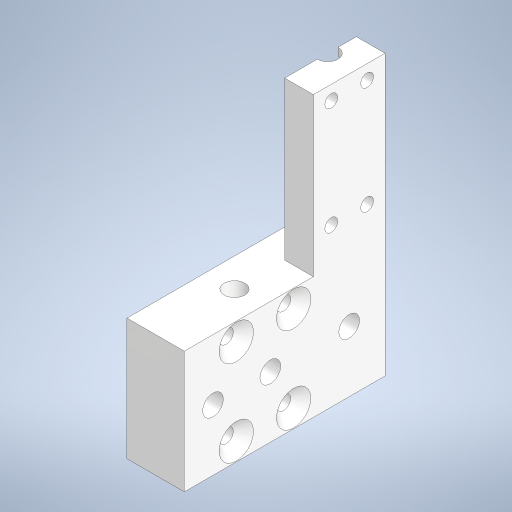
# Autodesk Inventor part: Z_probe_holder
Saved by Autodesk Inventor 2024.1 (Build 281209000, 209)
## iProperties
Created: 2023-10-06
Part Number: Z_probe_holder
Material: Generic
Document SubType Name: Modeling
Designer: l1534
Density: 1 g/cm^3
Appearance: White
Author: l1534
Autodesk Inventor part; units mm, degrees
ref_plane "YZ Plane" through (0, 0, 0) normal (1, 0, 0) x (0, 1, 0)
ref_plane "XZ Plane" through (0, 0, 0) normal (0, 1, 0) x (-1, 0, 0)
ref_plane "XY Plane" through (0, 0, 0) normal (0, 0, 1) x (1, 0, 0)
sketch "Sketch1" plane through (0, 0, 0) normal (1, 0, 0) x (0, 1, 0)
  line L0 (3.2139, -35.6679) -> (20.2139, -35.6679)
  line L1 (20.2139, -35.6679) -> (20.2139, -63.6679)
  line L2 (20.2139, -63.6679) -> (3.2139, -63.6679)
  line L3 (3.2139, -63.6679) -> (3.2139, -35.6679)
  point P0 (0, 0)
  dimension "d0" = 17
  dimension "d1" = 28
  constraints: 8 end point, 2 parallel, 1 horizontal, 1 perpendicular
  measures "d0" distance of L0.start L0.end
  measures "d1" distance of L0.end L1.end
extrude "Extrusion1" add sketch "Sketch1" along normal blind 8
sketch "Sketch2" plane through (8, 0, 0) normal (1, 0, 0) x (0, 0, -1)
  line L0 (63.6679, 3.2139) -> (63.6679, 20.2139) projected
  line L1 (63.6679, 20.2139) -> (53.6679, 20.2139)
  line L2 (53.6679, 20.2139) -> (53.6679, 42.2139)
  line L3 (53.6679, 42.2139) -> (63.6679, 42.2139)
  line L4 (63.6679, 42.2139) -> (63.6679, 20.2139)
  point P0 (0, 0)
  dimension "d4" = 10
  dimension "d5" = 22
  constraints: 8 end point, 2 parallel, 1 horizontal, 1 perpendicular
  measures "d4" distance of L2.end L3.end
  measures "d5" distance of L1.end L2.end
extrude "Extrusion2" add sketch "Sketch2" against normal up to surface (8 mm away)
sketch "Sketch3" plane through (8, 20.2139, -53.6679) normal (0, 0, 1) x (1, 0, 0)
  line L0 (-8, 0) -> (0, 0) projected
  line L1 (-8, -17) -> (-8, 22) projected
  line L2 (-4, 0) -> (-8, 0)
  line L3 (-8, 0) -> (-8, 22)
  line L4 (-8, 22) -> (-4, 22)
  line L5 (-4, 22) -> (-4, 0)
  point P0 (-8, -20.2139)
  dimension "d8" = 4
  constraints: 8 end point, 2 parallel, 1 horizontal, 1 midpoint, 1 perpendicular
  measures "d8" distance between parallel lines of L1 L5
extrude "Extrusion3" cut sketch "Sketch3" against normal through all
sketch "Sketch4" plane through (8, 0, 0) normal (1, 0, 0) x (0, 0, -1)
  circle A0 centre (42.9179, 5.7139) radius 1
  circle A1 centre (42.9179, 17.7139) radius 1
  circle A2 centre (50.9179, 5.7139) radius 1
  circle A3 centre (50.9179, 17.7139) radius 1
  line L0 (35.6679, 3.2139) -> (63.6679, 3.2139) projected
  line L1 (53.6679, 20.2139) -> (35.6679, 20.2139) projected
  line L2 (35.6679, 20.2139) -> (35.6679, 3.2139) projected
  point P0 (0, 0)
  dimension "d11" = 2
  dimension "d13" = 2
  dimension "d14" = 2
  dimension "d15" = 2
  dimension "d16" = 2.5
  dimension "d17" = 2.5
  dimension "d18" = 2.5
  dimension "d19" = 2.5
  dimension "d20" = 7.25
  dimension "d21" = 7.25
  dimension "d22" = 8
  dimension "d23" = 8
  constraints: 4 centre point
  measures "d11" diameter of A2
  measures "d13" diameter of A1
  measures "d14" diameter of A3
  measures "d15" diameter of A0
  measures "d16" distance from line of L0 A0.centre
  measures "d17" distance from line of L1 A1.centre
  measures "d18" distance from line of L1 A3.centre
  measures "d19" distance from line of L0 A2.centre
  measures "d20" distance from line of L2 A0.centre
  measures "d21" distance from line of L2 A1.centre
  measures "d22" distance of A0.centre A2.centre
  measures "d23" distance of A1.centre A3.centre
extrude "Extrusion4" cut sketch "Sketch4" against normal through all
sketch "Sketch5" plane through (0, 3.2139, -63.6679) normal (0, -1, 0) x (1, 0, 0)
  line L0 (4, 10) -> (4, 0) projected
  circle A0 centre (4, 4) radius 1.45
  circle A1 centre (4, 17) radius 1.45
  line L1 (8, 28) -> (8, 0) projected
  line L2 (0, 0) -> (8, 0) projected
  point P0 (0, 63.6679)
  dimension "d26" = 2.9
  dimension "d27" = 2.9
  dimension "d28" = 4
  dimension "d29" = 4
  dimension "d30" = 17
  constraints: 2 centre point, 1 point on line
  measures "d26" diameter of A1
  measures "d27" diameter of A0
  measures "d28" distance from line of L1 A1.centre
  measures "d29" distance from line of L2 A0.centre
  measures "d30" distance from line of L2 A1.centre
extrude "Extrusion5" cut sketch "Sketch5" against normal through all
chamfer "Chamfer1" distance 0.2 angle 45 2 edges at (2.55, 3.2139, -46.6679) (2.55, 3.2139, -59.6679)
sketch "Sketch7" plane through (8, 0, 0) normal (1, 0, 0) x (0, 0, -1)
  circle A0 centre (56.1679, 25.2139) radius 0.9
  circle A1 centre (56.1679, 40.2139) radius 0.9
  circle A2 centre (61.1679, 25.2139) radius 0.9
  circle A3 centre (61.1679, 40.2139) radius 0.9
  line L0 (53.6679, 42.2139) -> (53.6679, 20.2139) projected
  line L1 (63.6679, 3.2139) -> (63.6679, 42.2139) projected
  line L2 (63.6679, 42.2139) -> (53.6679, 42.2139) projected
  point P0 (0, 0)
  dimension "d36" = 1.8
  dimension "d37" = 1.8
  dimension "d38" = 1.8
  dimension "d39" = 1.8
  dimension "d40" = 2.5
  dimension "d41" = 2.5
  dimension "d42" = 2.5
  dimension "d43" = 2.5
  dimension "d44" = 15
  dimension "d45" = 15
  dimension "d46" = 2
  dimension "d47" = 2
  constraints: 4 centre point
  measures "d36" diameter of A0
  measures "d37" diameter of A2
  measures "d38" diameter of A1
  measures "d39" diameter of A3
  measures "d40" distance from line of L0 A0.centre
  measures "d41" distance from line of L1 A2.centre
  measures "d42" distance from line of L0 A1.centre
  measures "d43" distance from line of L1 A3.centre
  measures "d44" distance of A3.centre A2.centre
  measures "d45" distance of A1.centre A0.centre
  measures "d46" distance from line of L2 A1.centre
  measures "d47" distance from line of L2 A3.centre
extrude "Extrusion6" cut sketch "Sketch7" against normal through all
sketch "Sketch8" plane through (8, 0, 0) normal (1, 0, 0) x (0, 0, -1)
  circle A0 centre (39.6679, 11.7139) radius 1.45
  circle A1 centre (58.6679, 11.7139) radius 1.45
  circle A2 centre (47.6679, 11.7139) radius 1.45
  line L0 (53.6679, 20.2139) -> (35.6679, 20.2139) projected
  line L1 (35.6679, 3.2139) -> (63.6679, 3.2139) projected
  line L2 (63.6679, 3.2139) -> (63.6679, 42.2139) projected
  line L3 (35.6679, 20.2139) -> (35.6679, 3.2139) projected
  point P0 (0, 0)
  dimension "d53" = 8.5
  dimension "d54" = 8.5
  dimension "d55" = 8.5
  dimension "d56" = 2.9
  dimension "d57" = 2.9
  dimension "d58" = 2.9
  dimension "d59" = 5
  dimension "d60" = 16
  dimension "d61" = 4
  constraints: 3 centre point
  measures "d53" distance from line of L0 A0.centre
  measures "d54" distance from line of L0 A2.centre
  measures "d55" distance from line of L1 A1.centre
  measures "d56" diameter of A0
  measures "d57" diameter of A2
  measures "d58" diameter of A1
  measures "d59" distance from line of L2 A1.centre
  measures "d60" distance from line of L2 A2.centre
  measures "d61" distance from line of L3 A0.centre
extrude "Extrusion7" cut sketch "Sketch8" against normal through all
chamfer "Chamfer3" distance 1.4 angle 45 4 edges at (8, 5.7139, -41.9179) (8, 17.7139, -41.9179) (8, 17.7139, -49.9179) (8, 5.7139, -49.9179)
body "Solid1"
